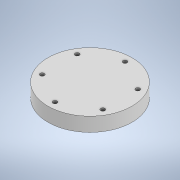
# Autodesk Inventor part: Base_To_First_Tilt_Attachment
Saved by Autodesk Inventor 2022.3 (Build 263350000, 350)
## iProperties
Created: 2022-05-27
Part Number: Base_To_First_Tilt_Attachment
Material: Generic
Document SubType Name: Modeling
Designer: Mlees
Density: 1 g/cm^3
Appearance: Default
Author: Mlees
Autodesk Inventor part; units mm, degrees
ref_plane "YZ Plane" through (0, 0, 0) normal (1, 0, 0) x (0, 1, 0)
ref_plane "XZ Plane" through (0, 0, 0) normal (0, 1, 0) x (-1, 0, 0)
ref_plane "XY Plane" through (0, 0, 0) normal (0, 0, 1) x (1, 0, 0)
sketch "Sketch1" plane through (0, 0, 0) normal (0, 1, 0) x (-1, 0, 0)
  circle A0 centre (0, 0) radius 12.75
  circle A1 centre (0, 0) radius 30
  dimension "d0" = 25.5
  dimension "d1" = 60
  constraints: 2 centre point, 2 coincident
  measures "d0" diameter of A0
  measures "d1" diameter of A1
extrude "Extrusion1" add sketch "Sketch1" along normal blind 7
sketch "Sketch2" plane through (0, 7, 0) normal (0, 1, 0) x (1, 0, 0)
  circle A0 centre (0, 0) radius 30
  constraints: 1 centre point, 1 coincident
extrude "Extrusion2" add sketch "Sketch2" along normal blind 3
sketch "Sketch3" plane through (0, 0, 0) normal (0, -1, 0) x (1, 0, 0)
  circle A0 centre (0, 0) radius 30 projected
  line L0 (0, 30) -> (0, 25)
  point P0 (-21.6506, 12.5)
  point P1 (-21.6506, -12.5)
  point P2 (0, -25)
  point P3 (21.6506, -12.5)
  point P4 (21.6506, 12.5)
  dimension "d6" = 5
  dimension "d9" = 360
  constraints: 2 end point, 1 coincident, 1 vertical, 1 vertical alignment, 8 other
  measures "d6" distance of L0.start L0.end
hole "Hole1" at (0, 0, 25) at (-21.6506, 0, 12.5) at (-21.6506, 0, -12.5) at (0, 0, -25) at (21.6506, 0, -12.5) at (21.6506, 0, 12.5) direction (0, 1, 0) diameter 3 end through all countersink diameter 5.5 countersink angle 90
body "Solid1"
